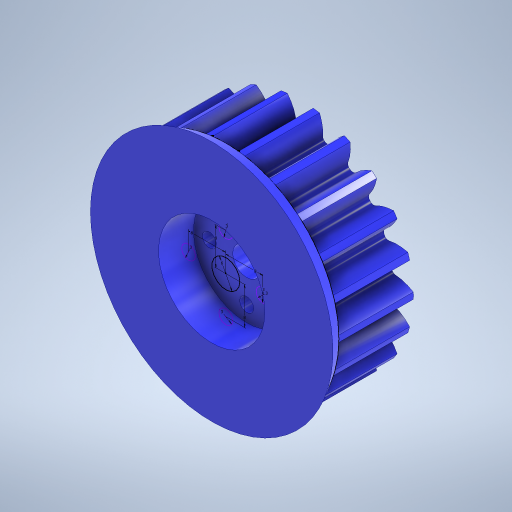
# Autodesk Inventor part: Шест
Saved by Autodesk Inventor 2024.2 (Build 282272000, 272)
## iProperties
Created: 2025-11-19
Part Number: Шест
Material: Generic
Document SubType Name: Modeling
Designer: Zakhar
Density: 1 g/cm^3
Appearance: Синий — малярная краска — глянцевая
Mass: 23.5328 g
Surface Area: 78.9857 cm^2
Volume: 23.5328 cm^3
Author: Zakhar
Autodesk Inventor part; units mm, degrees
ref_plane "YZ Plane" through (0, 0, 0) normal (1, 0, 0) x (0, 1, 0)
ref_plane "XZ Plane" through (0, 0, 0) normal (0, 1, 0) x (-1, 0, 0)
ref_plane "XY Plane" through (0, 0, 0) normal (0, 0, 1) x (1, 0, 0)
sketch "Sketch1" plane through (0, 0, 0) normal (0, 0, 1) x (1, 0, 0)
  spline S0 degree 3 poles (-2.7744, 24.0862) (-2.7058, 23.9974) (-2.5687, 23.8197) (-2.3726, 23.546) (-2.184, 23.2672) (-2.0043, 22.9825) (-1.834, 22.6921) (-1.6741, 22.3958) (-1.5256, 22.0937) (-1.4125, 21.8369) (-1.3296, 21.6283) (-1.2714, 21.4704) (-1.2177, 21.3108) (-1.1692, 21.1497) (-1.1262, 20.9869) (-1.0916, 20.8222) (-1.0673, 20.684) (-1.0401, 20.5751) (-1.0151, 20.4947) (-0.986, 20.4157) (-0.9529, 20.3383) (-0.9143, 20.2635) (-0.8705, 20.1915) (-0.8212, 20.1232) (-0.7662, 20.0595) (-0.7061, 20.0004) (-0.6403, 19.9477) (-0.5696, 19.9019) (-0.4951, 19.8625) (-0.4167, 19.8314) (-0.3354, 19.8094) (-0.2525, 19.794) (-0.1402, 19.7895) (0, 19.7924) (0.1402, 19.7895) (0.2525, 19.794) (0.3354, 19.8094) (0.4167, 19.8314) (0.4951, 19.8625) (0.5696, 19.9019) (0.6403, 19.9477) (0.7061, 20.0004) (0.7662, 20.0595) (0.8212, 20.1232) (0.8705, 20.1915) (0.9143, 20.2635) (0.9529, 20.3383) (0.986, 20.4157) (1.0151, 20.4947) (1.0401, 20.5751) (1.0673, 20.684) (1.0916, 20.8222) (1.1262, 20.9869) (1.1692, 21.1497) (1.2177, 21.3108) (1.2714, 21.4704) (1.3296, 21.6283) (1.4125, 21.8369) (1.5256, 22.0937) (1.6741, 22.3958) (1.834, 22.6921) (2.0043, 22.9825) (2.184, 23.2672) (2.3726, 23.546) (2.5687, 23.8197) (2.7058, 23.9974) (2.7744, 24.0862) knots 0 0 0 0 0.03366 0.06732 0.10098 0.13464 0.1683 0.201959 0.235618 0.269276 0.286107 0.302937 0.319767 0.336596 0.353426 0.370255 0.387082 0.395497 0.403912 0.412325 0.420739 0.429154 0.437568 0.445981 0.454393 0.462808 0.471222 0.479634 0.488046 0.49646 0.504872 0.513285 0.521697 0.538527 0.555357 0.563769 0.572182 0.580593 0.589007 0.59742 0.605831 0.614246 0.62266 0.631073 0.639486 0.6479 0.656314 0.664729 0.673142 0.681557 0.689971 0.706799 0.723628 0.740457 0.757287 0.774117 0.790947 0.807777 0.841436 0.875095 0.908754 0.942414 0.976073 1.009733 1.043394 1.077054 1.077054 1.077054 1.077054
  circle A0 centre (0, 0) radius 19.7912 construction
  circle A1 centre (0, 0) radius 20.6732 construction
  circle A2 centre (0, 0) radius 22 construction
  circle A3 centre (0, 0) radius 24.2454
  circle A4 centre (0, 0) radius 3
  circle A5 centre (0, -8) radius 1.5
  circle A6 centre (8, 0) radius 1.5
  circle A7 centre (0, 8) radius 1.5
  circle A8 centre (8, 0) radius 1.5
  circle A9 centre (-8, 0) radius 1.5
  point P0 (-2.5703, 23.8185)
  point P1 (-2.3739, 23.5452)
  point P2 (-2.1855, 23.2662)
  point P3 (-2.0059, 22.9815)
  point P4 (-1.8357, 22.6911)
  point P5 (-1.676, 22.3949)
  point P6 (-1.5277, 22.0927)
  point P7 (-1.3924, 21.7845)
  point P8 (-1.3302, 21.6281)
  point P9 (-1.2722, 21.4701)
  point P10 (-1.2186, 21.3106)
  point P11 (-1.1701, 21.1494)
  point P12 (-1.1276, 20.9866)
  point P13 (-1.0925, 20.822)
  point P14 (-1.0599, 20.6569)
  point P15 (-1.0393, 20.5753)
  point P16 (-1.0144, 20.4949)
  point P17 (-0.9853, 20.416)
  point P18 (-0.952, 20.3387)
  point P19 (-0.9134, 20.2639)
  point P20 (-0.8696, 20.1921)
  point P21 (-0.8202, 20.124)
  point P22 (-0.7653, 20.0603)
  point P23 (-0.7051, 20.0015)
  point P24 (-0.6395, 19.9489)
  point P25 (-0.5689, 19.903)
  point P26 (-0.4945, 19.8639)
  point P27 (-0.4162, 19.8329)
  point P28 (-0.3352, 19.8105)
  point P29 (-0.2523, 19.796)
  point P30 (-0.1683, 19.7912)
  point P31 (0, 19.7912)
  point P32 (0.1683, 19.7912)
  point P33 (0.2523, 19.796)
  point P34 (0.3352, 19.8105)
  point P35 (0.4162, 19.8329)
  point P36 (0.4945, 19.8639)
  point P37 (0.5689, 19.903)
  point P38 (0.6395, 19.9489)
  point P39 (0.7051, 20.0015)
  point P40 (0.7653, 20.0603)
  point P41 (0.8202, 20.124)
  point P42 (0.8696, 20.1921)
  point P43 (0.9134, 20.2639)
  point P44 (0.952, 20.3387)
  point P45 (0.9853, 20.416)
  point P46 (1.0144, 20.4949)
  point P47 (1.0393, 20.5753)
  point P48 (1.0599, 20.6569)
  point P49 (1.0925, 20.822)
  point P50 (1.1276, 20.9866)
  point P51 (1.1701, 21.1494)
  point P52 (1.2186, 21.3106)
  point P53 (1.2722, 21.4701)
  point P54 (1.3302, 21.6281)
  point P55 (1.3924, 21.7845)
  point P56 (1.5277, 22.0927)
  point P57 (1.676, 22.3949)
  point P58 (1.8357, 22.6911)
  point P59 (2.0059, 22.9815)
  point P60 (2.1855, 23.2662)
  point P61 (2.3739, 23.5452)
  point P62 (2.5703, 23.8185)
  dimension "d9" = 6
  dimension "d10" = 3
  dimension "d11" = 3
  dimension "d12" = 3
  dimension "d13" = 3
  dimension "d14" = 8
  dimension "d15" = 8
  dimension "d16" = 8
  dimension "d17" = 8
  dimension "d18" = 3
  constraints: 10 centre point, 2 coincident, 2 point on circle, 135 other
  measures "d9" diameter of A4
  measures "d10" diameter of A6
  measures "d11" diameter of A7
  measures "d12" diameter of A5
  measures "d13" diameter of A8
  measures "d14" distance of A7.centre A1.centre
  measures "d15" distance of A5.centre A0.centre
  measures "d16" distance of A6.centre point (0, 0)
  measures "d17" distance of A9.centre point (0, 0)
  measures "d18" diameter of A9
extrude "Выдавливание1" add sketch "Sketch1" against normal blind 16 contours A3 S0 | S0 A3 | A4 | A5 | A6 | A7 | A9
extrude "Выдавливание2" cut sketch "Sketch1" against normal through all fills toward (0, 19.8412) open curves S0
pattern_circular "Круговой массив1" count 22 over 360 about axis through (0, 0, 0) along (0, 0, -1) of "Выдавливание2"
extrude "Выдавливание3" cut sketch "Sketch1" against normal up to surface (16 mm away) contours A4 | A5 | A6 | A7 | A9
ref_plane "РабПлоскость1" through (0, 0, 3) normal (0, 0, 1) x (1, 0, 0)
sketch "Эскиз2" plane through (0, 0, 3) normal (0, 0, 1) x (1, 0, 0)
  circle A0 centre (0, 0) radius 26
  dimension "d23" = 52
  constraints: 1 centre point, 1 coincident
  measures "d23" diameter of A0
sketch "Эскиз3" plane through (0, 0, 0) normal (0, 0, 1) x (1, 0, 0)
  circle A0 centre (0, 0) radius 24.2454
  circle A1 centre (0, 0) radius 24.2454 projected
  constraints: 1 centre point, 1 coincident, 1 concentric
loft "Лофт1" add profiles "Эскиз3", "Эскиз2"
sketch "Эскиз4" plane through (0, 0, 3) normal (0, 0, 1) x (1, 0, 0)
  circle A0 centre (0, 0) radius 3 projected
  circle A1 centre (-8, 0) radius 1.5 projected
  circle A2 centre (0, -8) radius 1.5 projected
  circle A3 centre (8, 0) radius 1.5 projected
  circle A4 centre (0, 8) radius 1.5 projected
  circle A5 centre (0, 0) radius 11.4
  dimension "d28" = 22.8
  constraints: 1 centre point, 1 coincident
  measures "d28" diameter of A5
extrude "Выдавливание4" cut sketch "Эскиз4" against normal blind 7.5
extrude "Выдавливание5" cut sketch "Sketch1" along normal blind 3 contours A4 | A5 | A6 | A7 | A9
ref_plane "РабПлоскость2" through (0, 0, -19) normal (0, 0, -1) x (-1, 0, 0)
equation "\"d0\" = Ширина_грани"
equation "\"Модуль\" = 2"
equation "\"Угол_зацепления\" = 20deg"
equation "\"Зазор_профиля_зуба\" = 0.25"
equation "\"Радиус_закругления_зуба\" = 0.35"
equation "\"Диаметр_головки\" = 48.49088"
equation "\"Диаметр_впадин\" = 39.58247"
equation "\"Основной_диаметр\" = 41.34648"
equation "\"Средний_диаметр\" = 44"
equation "\"Ширина_грани\" = 16"
equation "\"Коэффициент_смещения\" = 0.145617"
equation "\"Изменение_высоты_головки_зуба\" = 0.022898"
equation "\"Окружной_шаг\" = 6.283185"
equation "\"Общий_сдвиг_инструмента\" = 0.29123"
equation "\"Внутренний\" = 0"
